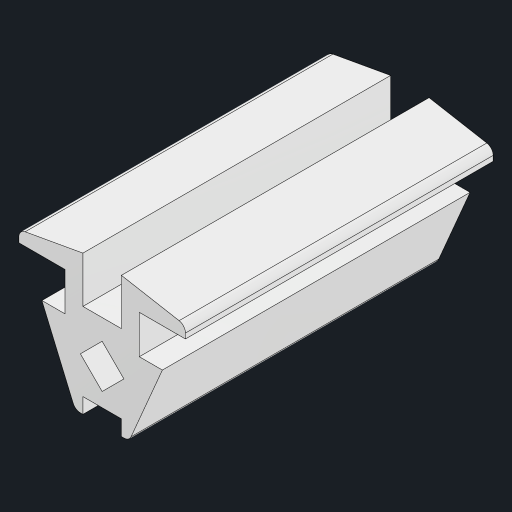
# Autodesk Inventor part: TailRod_N_o
Saved by Autodesk Inventor 2023 (Build 270158000, 158)
## iProperties
Created: 2022-05-26
Part Number: TailRod_N_o
Material: ABS プラスチック
Document SubType Name: Modeling
Designer: neko2
Density: 1.06 g/cm^3
Appearance: 滑らか - 白
Mass: 5.90992 g
Surface Area: 47.4859 cm^2
Volume: 5.5754 cm^3
Author: neko2
Autodesk Inventor part; units mm, degrees
ref_plane "YZ Plane" through (0, 0, 0) normal (1, 0, 0) x (0, 1, 0)
ref_plane "XZ Plane" through (0, 0, 0) normal (0, 1, 0) x (-1, 0, 0)
ref_plane "XY Plane" through (0, 0, 0) normal (0, 0, 1) x (1, 0, 0)
sketch "スケッチ1" plane through (0, 0, 0) normal (0, 0, 1) x (1, 0, 0)
  line L0 (0, 18.2674) -> (0, -9.7942)
  line L1 (0, -4.65) -> (-2.5, -4.65)
  line L2 (-2.5, -4.65) -> (-2.5, -6.65)
  line L3 (-2.5, -6.65) -> (-3.5, -6.65)
  line L4 (-10.8284, 8.5) -> (-4.8284, 8.5)
  line L5 (-4.8284, 8.5) -> (-4.8284, 3.5)
  line L6 (-4.8284, 3.5) -> (-7.8284, 3.5)
  line L7 (-7.8284, 3.5) -> (-3.5, -6.65)
  line L8 (-10.8284, 8.5) -> (-10.8284, 10)
  line L9 (-10.8284, 10) -> (-2.5, 11.5)
  line L10 (-2.5, 11.5) -> (-2.5, 5.5)
  line L11 (-2.5, 5.5) -> (0, 5.5)
  line L12 (0, -4.65) -> (2.5, -4.65)
  line L13 (2.5, -4.65) -> (2.5, -6.65)
  line L14 (2.5, -6.65) -> (3.5, -6.65)
  line L15 (10.8284, 8.5) -> (4.8284, 8.5)
  line L16 (4.8284, 8.5) -> (4.8284, 3.5)
  line L17 (4.8284, 3.5) -> (7.8284, 3.5)
  line L18 (7.8284, 3.5) -> (3.5, -6.65)
  line L19 (10.8284, 8.5) -> (10.8284, 10)
  line L20 (10.8284, 10) -> (2.5, 11.5)
  line L21 (2.5, 11.5) -> (2.5, 5.5)
  line L22 (2.5, 5.5) -> (0, 5.5)
  line L23 (-2.8284, 0) -> (0, 2.8284)
  line L24 (0, 2.8284) -> (2.8284, 0)
  line L25 (2.8284, 0) -> (0, -2.8284)
  line L26 (0, -2.8284) -> (-2.8284, 0)
  point P0 (0, 0)
  point P1 (0, 3.5)
  point P2 (0, -2.65)
  point P3 (2.8284, 0)
  dimension "d23" = 2
  dimension "d31" = 1
  dimension "d33" = 2
  dimension "d34" = 6
  dimension "d35" = 3
  dimension "d39" = 5
  dimension "d41" = 3
  dimension "d42" = 5
  dimension "d43" = 5
  dimension "d44" = 2
  dimension "d45" = 1.5
  dimension "d46" = 2
  dimension "d50" = 4
  dimension "d51" = 3.5
  constraints: 54 end point, 11 symmetric about line, 7 perpendicular, 6 point on line, 3 parallel, 2 horizontal, 2 horizontal alignment, 2 vertical, 1 coincident, 1 vertical alignment
  measures "d23" distance of point (0, -2.65) L1.start
  measures "d31" distance of L2.end L3.end
  measures "d33" distance of L1.end L2.end
  measures "d34" distance of L4.start L4.end
  measures "d35" distance of L5.end L6.end
  measures "d39" distance of L4.end L5.end
  measures "d41" vertical distance of L9.end L4.end
  measures "d42" diameter of L10.end L0
  measures "d43" diameter of L1.end L0
  measures "d44" distance of point (0, 3.5) L11.end
  measures "d45" distance of L4.start L8.end
  measures "d46" horizontal distance of point (-2.828, 0) L5.end
  measures "d50" distance of L23.end L24.end
  measures "d51" distance from line of point (0, 0) L17
extrude "押し出し1" add sketch "スケッチ1" along normal blind 40 contours L22 L21 L20 L19 L15 L16 L17 L18 L14 L13 L12 L0 L25 L24 | L0 L23 L26 L1 L2 L3 L7 L6 L5 L4 L8 L9 L10 L11
fillet "フィレット2" radius 1 4 edges at (-3.5, -6.65, 20) (3.5, -6.65, 20) (10.8284, 10, 20) (-10.8284, 10, 20)
